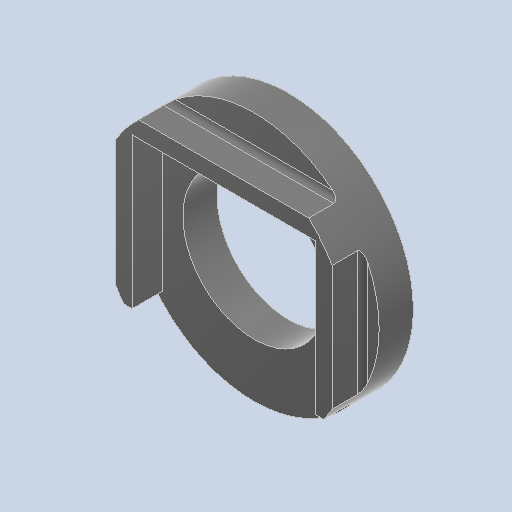
# Autodesk Inventor part: connectpart2
Saved by Autodesk Inventor 2024.3 (Build 283343010, 343A)
## iProperties
Created: 2025-06-26
Part Number: connectpart2
Material: 一般
Document SubType Name: Modeling
Designer: kshau
Density: 1 g/cm^3
Appearance: 滑らか - 黒
Author: kshau
Autodesk Inventor part; units mm, degrees
ref_plane "YZ Plane" through (0, 0, 0) normal (1, 0, 0) x (0, 1, 0)
ref_plane "XZ Plane" through (0, 0, 0) normal (0, 1, 0) x (-1, 0, 0)
ref_plane "XY Plane" through (0, 0, 0) normal (0, 0, 1) x (1, 0, 0)
sketch "スケッチ1" plane through (0, 0, 0) normal (0, 0, 1) x (1, 0, 0)
  circle A0 centre (0, 0) radius 23
  dimension "d0" = 46
  constraints: 1 centre point, 1 coincident
  measures "d0" diameter of A0
extrude "押し出し1" add sketch "スケッチ1" along normal blind 6.3
sketch "スケッチ2" plane through (0, 0, 6.3) normal (0, 0, 1) x (1, 0, 0)
  line L0 (0, 0) -> (16.85, 0)
  line L1 (16.85, 0) -> (16.85, 13.85)
  line L2 (16.85, 13.85) -> (0, 13.85)
  line L3 (0, 13.85) -> (0, 0)
  line L4 (0, 0) -> (-16.85, 0)
  line L5 (-16.85, 0) -> (-16.85, 13.85)
  line L6 (-16.85, 13.85) -> (0, 13.85)
  line L7 (-19.95, -13.85) -> (19.95, -13.85)
  line L8 (19.95, -13.85) -> (19.95, 16.85)
  line L9 (19.95, 16.85) -> (-19.95, 16.85)
  line L10 (-19.95, 16.85) -> (-19.95, -13.85)
  line L11 (-16.85, 0) -> (-16.85, -13.85)
  line L12 (16.85, 0) -> (16.85, -13.85)
  circle A0 centre (0, 0) radius 23
  point P0 (18.3624, -13.85)
  point P1 (19.95, -11.4454)
  point P2 (19.95, 11.4454)
  point P3 (15.655, 16.85)
  point P4 (-15.655, 16.85)
  point P5 (-19.95, 11.4454)
  point P6 (-19.95, -11.4454)
  point P7 (-18.3624, -13.85)
  dimension "d3" = 13.85
  dimension "d4" = 16.85
  dimension "d5" = 3
  dimension "d6" = 3.1
  dimension "d8" = 3.1
  dimension "d9" = 30.7
  dimension "d10" = 46
  constraints: 26 end point, 4 parallel, 4 perpendicular, 2 horizontal, 2 point on line, 2 symmetric about line, 1 centre point, 1 coincident
  measures "d3" distance between parallel lines of L0 L2
  measures "d4" distance between parallel lines of L3 L1
  measures "d5" distance between parallel lines of L6 L9
  measures "d6" distance between parallel lines of L5 L10
  measures "d8" distance between parallel lines of L1 L8
  measures "d9" distance of L9.end L7.start
  measures "d10" diameter of A0
extrude "押し出し2" add sketch "スケッチ2" along normal blind 5.6 contours L1 L2 L6 L5 L11 L7 A0 L10 L9 L8 L12
sketch "スケッチ3" plane through (0, 0, 6.3) normal (0, 0, 1) x (1, 0, 0)
  circle A0 centre (0, 0) radius 13.1
  dimension "d13" = 26.2
  constraints: 1 centre point, 1 coincident
  measures "d13" diameter of A0
extrude "押し出し3" cut sketch "スケッチ3" against normal blind 7
sketch "スケッチ4" plane through (0, 0, 0) normal (0, 0, -1) x (-1, 0, 0)
  circle A0 centre (0, 0) radius 19.5
  dimension "d16" = 39
  constraints: 1 centre point, 1 coincident
  measures "d16" diameter of A0
extrude "押し出し4" [suppressed]
fillet "フィレット1" radius 1 3 edges at (0, 16.85, 6.3) (19.95, 0, 6.3) (-19.95, 0, 6.3)
